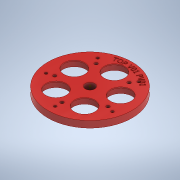
# Autodesk Inventor part: filterHolderBackPiece
Saved by Autodesk Inventor 2022.2 (Build 262287000, 287)
## iProperties
Created: 2020-04-12
Part Number: filterHolderBackPiece
Material: PBT Plastic
Document SubType Name: Modeling
Designer: robst
Density: 1.31 g/cm^3
Appearance: Orange-Red
wheelOuterDiameter: 4.501 in
wheelFilterDiameter: 2.611 in
filterThreadDiameter: 1.100 in
numberOfFilters: 5.000 ul
d5: 360.00 deg
distanceBetweenFilters: 0.500 in
distanceFromFilterToEdge: 0.375 in
wheelFilterCircumference: 8.200 in
filterDiameter: 1.140 in
Author: robst
Autodesk Inventor part; units mm, degrees
ref_plane "YZ Plane" through (0, 0, 0) normal (1, 0, 0) x (0, 1, 0)
ref_plane "XZ Plane" through (0, 0, 0) normal (0, 1, 0) x (-1, 0, 0)
ref_plane "XY Plane" through (0, 0, 0) normal (0, 0, 1) x (1, 0, 0)
sketch "Sketch1" plane through (0, 0, 0) normal (0, 1, 0) x (-1, 0, 0)
  circle A0 centre (0, 0) radius 57.1686
  circle A1 centre (0, 0) radius 33.1656 construction
  circle A2 centre (0, -33.1656) radius 13.97
  circle A3 centre (31.5424, -10.2487) radius 13.97
  circle A4 centre (19.4943, 26.8315) radius 13.97
  circle A5 centre (-19.4943, 26.8315) radius 13.97
  circle A6 centre (-31.5424, -10.2487) radius 13.97
  dimension "wheelFilterDiameter" = 66.3312
  dimension "wheelOuterDiameter" = 114.3372
  dimension "filterThreadDiameter" = 27.94
  dimension "d5" = 360
  constraints: 6 centre point, 2 coincident, 1 vertical alignment, 13 other
  measures "wheelOuterDiameter" diameter of A0
  measures "filterThreadDiameter" diameter of A2
extrude "Extrusion5" add sketch "Sketch1" against normal blind 8.89
sketch "Sketch5" plane through (0, 0, 0) normal (0, 1, 0) x (1, 0, 0)
  arc A0 (35.921, 35.921) -> (0, 50.8) centre (0, 0) ccw construction
  line L0 (0, 0) -> (0, 50.8) construction
  line L1 (0, 0) -> (35.921, 35.921) construction
  line L2 (0, 0) -> (50.8, 0) construction
  line L3 (-13.9692, 45.6649) -> (-15.4973, 50.8179)
  line L4 (-15.4973, 50.8179) -> (-17.4581, 50.2364)
  line L5 (-17.4581, 50.2364) -> (-17.6631, 50.9279)
  line L6 (-17.6631, 50.9279) -> (-12.9648, 52.3211)
  line L7 (-12.9648, 52.3211) -> (-12.7598, 51.6296)
  line L8 (-12.7598, 51.6296) -> (-14.7205, 51.0482)
  line L9 (-14.7205, 51.0482) -> (-13.1925, 45.8952)
  line L10 (-13.1925, 45.8952) -> (-13.9692, 45.6649)
  spline S0 degree 2 poles (-7.3189, 52.6818) (-6.9078, 52.3431) (-6.322, 51.2426) (-6.1896, 50.4935) knots 0 0 0 1 2 2 2
  spline S1 degree 2 poles (-6.1896, 50.4935) (-6.0606, 49.7638) (-6.2213, 48.5163) (-6.5011, 48.0555) knots 0 0 0 1 2 2 2
  spline S2 degree 2 poles (-6.5011, 48.0555) (-6.7968, 47.5718) (-7.7041, 47.0001) (-8.2927, 46.896) knots 0 0 0 1 2 2 2
  spline S3 degree 2 poles (-8.2927, 46.896) (-8.9008, 46.7885) (-9.9468, 47.03) (-10.3733, 47.371) knots 0 0 0 1 2 2 2
  spline S4 degree 2 poles (-10.3733, 47.371) (-10.7892, 47.7088) (-11.3662, 48.8158) (-11.4969, 49.5553) knots 0 0 0 1 2 2 2
  spline S5 degree 2 poles (-11.4969, 49.5553) (-11.6302, 50.3093) (-11.4585, 51.5235) (-11.1862, 51.9981) knots 0 0 0 1 2 2 2
  spline S6 degree 2 poles (-11.1862, 51.9981) (-10.9065, 52.4589) (-10.0018, 53.0452) (-9.3986, 53.1519) knots 0 0 0 1 2 2 2
  spline S7 degree 2 poles (-9.3986, 53.1519) (-8.7857, 53.2602) (-7.7273, 53.0059) (-7.3189, 52.6818) knots 0 0 0 1 2 2 2
  spline S8 degree 2 poles (-7.0214, 50.3464) (-7.1263, 50.9399) (-7.5467, 51.8137) (-7.8335, 52.0741) knots 0 0 0 1 2 2 2
  spline S9 degree 2 poles (-7.8335, 52.0741) (-8.1269, 52.3433) (-8.8533, 52.5359) (-9.2716, 52.462) knots 0 0 0 1 2 2 2
  spline S10 degree 2 poles (-9.2716, 52.462) (-9.7046, 52.3854) (-10.3031, 51.9686) (-10.4945, 51.6037) knots 0 0 0 1 2 2 2
  spline S11 degree 2 poles (-10.4945, 51.6037) (-10.6786, 51.2551) (-10.7682, 50.2861) (-10.665, 49.7023) knots 0 0 0 1 2 2 2
  spline S12 degree 2 poles (-10.665, 49.7023) (-10.4561, 48.5202) (-9.2418, 47.4406) (-8.41, 47.5876) knots 0 0 0 1 2 2 2
  spline S13 degree 2 poles (-8.41, 47.5876) (-7.5781, 47.7347) (-6.8125, 49.1643) (-7.0214, 50.3464) knots 0 0 0 1 2 2 2
  spline S14 degree 2 poles (-1.2006, 52.0412) (-1.1751, 51.6469) (-1.4102, 50.9188) (-1.6457, 50.6561) knots 0 0 0 1 2 2 2
  spline S15 degree 2 poles (-1.6457, 50.6561) (-1.9412, 50.3251) (-2.7733, 49.9495) (-3.424, 49.9075) knots 0 0 0 1 2 2 2
  line L11 (-3.424, 49.9075) -> (-4.1093, 49.8632)
  line L12 (-4.1093, 49.8632) -> (-3.9627, 47.5955)
  line L13 (-3.9627, 47.5955) -> (-4.7711, 47.5433)
  line L14 (-4.7711, 47.5433) -> (-5.1644, 53.6266)
  line L15 (-5.1644, 53.6266) -> (-3.6362, 53.7253)
  spline S16 degree 2 poles (-3.6362, 53.7253) (-3.0939, 53.7604) (-2.3232, 53.632) (-2.0193, 53.4487) knots 0 0 0 1 2 2 2
  spline S17 degree 2 poles (-2.0193, 53.4487) (-1.6642, 53.239) (-1.2335, 52.549) (-1.2006, 52.0412) knots 0 0 0 1 2 2 2
  spline S18 degree 2 poles (-2.042, 51.9621) (-2.0624, 52.2776) (-2.3093, 52.727) (-2.5407, 52.8605) knots 0 0 0 1 2 2 2
  spline S19 degree 2 poles (-2.5407, 52.8605) (-2.7412, 52.9763) (-3.2606, 53.0467) (-3.6402, 53.0221) knots 0 0 0 1 2 2 2
  line L16 (-3.6402, 53.0221) -> (-4.3106, 52.9788)
  line L17 (-4.3106, 52.9788) -> (-4.1539, 50.5534)
  line L18 (-4.1539, 50.5534) -> (-3.6017, 50.589)
  spline S20 degree 2 poles (-3.6017, 50.589) (-3.1088, 50.6209) (-2.5126, 50.8179) (-2.3288, 51.0377) knots 0 0 0 1 2 2 2
  spline S21 degree 2 poles (-2.3288, 51.0377) (-2.1582, 51.2318) (-2.0232, 51.6712) (-2.042, 51.9621) knots 0 0 0 1 2 2 2
  line L19 (7.4234, 53.3925) -> (4.7744, 47.5144)
  line L20 (4.7744, 47.5144) -> (3.9037, 47.5945)
  line L21 (3.9037, 47.5945) -> (2.3713, 53.8572)
  line L22 (2.3713, 53.8572) -> (3.2371, 53.7775)
  line L23 (3.2371, 53.7775) -> (4.4558, 48.5806)
  line L24 (4.4558, 48.5806) -> (6.6019, 53.4681)
  line L25 (6.6019, 53.4681) -> (7.4234, 53.3925)
  spline S22 degree 2 poles (11.6414, 49.4866) (11.3274, 47.8769) (10.0975, 46.5515) (9.1229, 46.7416) knots 0 0 0 1 2 2 2
  spline S23 degree 2 poles (9.1229, 46.7416) (8.1338, 46.9345) (7.5075, 48.6522) (7.8149, 50.228) knots 0 0 0 1 2 2 2
  spline S24 degree 2 poles (7.8149, 50.228) (8.1308, 51.8475) (9.3589, 53.1632) (10.3383, 52.9721) knots 0 0 0 1 2 2 2
  spline S25 degree 2 poles (10.3383, 52.9721) (11.3226, 52.7801) (11.946, 51.0479) (11.6414, 49.4866) knots 0 0 0 1 2 2 2
  spline S26 degree 2 poles (10.2579, 47.864) (10.432, 48.1371) (10.7067, 49.0297) (10.8269, 49.6455) knots 0 0 0 1 2 2 2
  spline S27 degree 2 poles (10.8269, 49.6455) (10.947, 50.2613) (11.0269, 51.1869) (10.9652, 51.516) knots 0 0 0 1 2 2 2
  spline S28 degree 2 poles (10.9652, 51.516) (10.9036, 51.8451) (10.5433, 52.2426) (10.2087, 52.3078) knots 0 0 0 1 2 2 2
  spline S29 degree 2 poles (10.2087, 52.3078) (9.8741, 52.3731) (9.3811, 52.1421) (9.1936, 51.8515) knots 0 0 0 1 2 2 2
  spline S30 degree 2 poles (9.1936, 51.8515) (9.0128, 51.5697) (8.7439, 50.6558) (8.6295, 50.0691) knots 0 0 0 1 2 2 2
  spline S31 degree 2 poles (8.6295, 50.0691) (8.5065, 49.4388) (8.4195, 48.58) (8.4813, 48.2257) knots 0 0 0 1 2 2 2
  spline S32 degree 2 poles (8.4813, 48.2257) (8.5371, 47.8927) (8.9034, 47.474) (9.2525, 47.4059) knots 0 0 0 1 2 2 2
  spline S33 degree 2 poles (9.2525, 47.4059) (9.5822, 47.3415) (10.0752, 47.5725) (10.2579, 47.864) knots 0 0 0 1 2 2 2
  line L26 (15.1243, 45.3222) -> (12.2732, 46.168)
  line L27 (12.2732, 46.168) -> (12.4502, 46.7647)
  line L28 (12.4502, 46.7647) -> (13.5111, 46.45)
  line L29 (13.5111, 46.45) -> (14.673, 50.3667)
  line L30 (14.673, 50.3667) -> (13.6121, 50.6814)
  line L31 (13.6121, 50.6814) -> (13.7708, 51.2166)
  spline S34 degree 2 poles (13.7708, 51.2166) (14.3723, 51.0382) (15.0418, 51.2106) (15.2202, 51.6729) knots 0 0 0 1 2 2 2
  line L32 (15.2202, 51.6729) -> (15.8264, 51.4931)
  line L33 (15.8264, 51.4931) -> (14.2641, 46.2266)
  line L34 (14.2641, 46.2266) -> (15.3013, 45.9189)
  line L35 (15.3013, 45.9189) -> (15.1243, 45.3222)
  spline S35 degree 2 poles (24.0801, 46.1507) (23.9119, 45.793) (23.3545, 45.269) (23.0214, 45.1527) knots 0 0 0 1 2 2 2
  spline S36 degree 2 poles (23.0214, 45.1527) (22.6029, 45.0055) (21.6928, 45.0785) (21.1027, 45.3559) knots 0 0 0 1 2 2 2
  line L36 (21.1027, 45.3559) -> (20.4813, 45.648)
  line L37 (20.4813, 45.648) -> (19.5145, 43.5915)
  line L38 (19.5145, 43.5915) -> (18.7813, 43.9362)
  line L39 (18.7813, 43.9362) -> (21.3747, 49.453)
  line L40 (21.3747, 49.453) -> (22.7606, 48.8015)
  spline S37 degree 2 poles (22.7606, 48.8015) (23.2524, 48.5703) (23.8652, 48.0857) (24.0428, 47.7785) knots 0 0 0 1 2 2 2
  spline S38 degree 2 poles (24.0428, 47.7785) (24.2525, 47.4233) (24.2965, 46.6111) (24.0801, 46.1507) knots 0 0 0 1 2 2 2
  spline S39 degree 2 poles (23.3051, 46.4877) (23.4396, 46.7738) (23.4404, 47.2865) (23.3023, 47.5152) knots 0 0 0 1 2 2 2
  spline S40 degree 2 poles (23.3023, 47.5152) (23.1825, 47.7134) (22.7617, 48.0259) (22.4175, 48.1877) knots 0 0 0 1 2 2 2
  line L41 (22.4175, 48.1877) -> (21.8095, 48.4735)
  line L42 (21.8095, 48.4735) -> (20.7755, 46.2739)
  line L43 (20.7755, 46.2739) -> (21.2762, 46.0385)
  spline S41 degree 2 poles (21.2762, 46.0385) (21.7233, 45.8284) (22.3404, 45.7129) (22.6075, 45.8167) knots 0 0 0 1 2 2 2
  spline S42 degree 2 poles (22.6075, 45.8167) (22.8507, 45.9043) (23.1811, 46.2239) (23.3051, 46.4877) knots 0 0 0 1 2 2 2
  line L44 (29.8707, 44.8732) -> (24.9322, 40.7284)
  line L45 (24.9322, 40.7284) -> (24.1826, 41.1786)
  line L46 (24.1826, 41.1786) -> (25.5215, 47.4855)
  line L47 (25.5215, 47.4855) -> (26.2669, 47.0378)
  line L48 (26.2669, 47.0378) -> (25.108, 41.8272)
  line L49 (25.108, 41.8272) -> (29.1635, 45.298)
  line L50 (29.1635, 45.298) -> (29.8707, 44.8732)
  spline S43 degree 2 poles (31.9744, 39.5232) (30.9925, 38.2095) (29.3091, 37.5496) (28.5137, 38.1441) knots 0 0 0 1 2 2 2
  spline S44 degree 2 poles (28.5137, 38.1441) (27.7065, 38.7474) (27.8882, 40.5666) (28.8493, 41.8526) knots 0 0 0 1 2 2 2
  spline S45 degree 2 poles (28.8493, 41.8526) (29.8371, 43.1743) (31.5146, 43.8262) (32.3139, 43.2288) knots 0 0 0 1 2 2 2
  spline S46 degree 2 poles (32.3139, 43.2288) (33.1172, 42.6285) (32.9267, 40.7974) (31.9744, 39.5232) knots 0 0 0 1 2 2 2
  spline S47 degree 2 poles (30.0235, 38.6624) (30.2989, 38.8328) (30.934, 39.5175) (31.3096, 40.0201) knots 0 0 0 1 2 2 2
  spline S48 degree 2 poles (31.3096, 40.0201) (31.6852, 40.5226) (32.1591, 41.3217) (32.2465, 41.6449) knots 0 0 0 1 2 2 2
  spline S49 degree 2 poles (32.2465, 41.6449) (32.3338, 41.9682) (32.1818, 42.4827) (31.9088, 42.6867) knots 0 0 0 1 2 2 2
  spline S50 degree 2 poles (31.9088, 42.6867) (31.6357, 42.8908) (31.0913, 42.8968) (30.7962, 42.7165) knots 0 0 0 1 2 2 2
  spline S51 degree 2 poles (30.7962, 42.7165) (30.511, 42.5411) (29.872, 41.8346) (29.5141, 41.3558) knots 0 0 0 1 2 2 2
  spline S52 degree 2 poles (29.5141, 41.3558) (29.1297, 40.8414) (28.6784, 40.1055) (28.5802, 39.7596) knots 0 0 0 1 2 2 2
  spline S53 degree 2 poles (28.5802, 39.7596) (28.4859, 39.4353) (28.634, 38.8991) (28.9189, 38.6862) knots 0 0 0 1 2 2 2
  spline S54 degree 2 poles (28.9189, 38.6862) (29.188, 38.4851) (29.7324, 38.4791) (30.0235, 38.6624) knots 0 0 0 1 2 2 2
  line L51 (33.3036, 34.2596) -> (31.1025, 36.2594)
  line L52 (31.1025, 36.2594) -> (31.5211, 36.7201)
  line L53 (31.5211, 36.7201) -> (32.3401, 35.976)
  line L54 (32.3401, 35.976) -> (35.0874, 38.9997)
  line L55 (35.0874, 38.9997) -> (34.2684, 39.7438)
  line L56 (34.2684, 39.7438) -> (34.6438, 40.157)
  spline S55 degree 2 poles (34.6438, 40.157) (35.1081, 39.7351) (35.786, 39.5997) (36.1475, 39.9388) knots 0 0 0 1 2 2 2
  line L57 (36.1475, 39.9388) -> (36.6155, 39.5136)
  line L58 (36.6155, 39.5136) -> (32.9214, 35.4478)
  line L59 (32.9214, 35.4478) -> (33.7221, 34.7203)
  line L60 (33.7221, 34.7203) -> (33.3036, 34.2596)
  dimension "d25" = 101.6
  dimension "d26" = 45
  constraints: 6 end point, 2 point on circle, 1 centre point, 1 coincident, 1 equal length, 1 horizontal, 1 vertical, 1 other
  measures "d25" diameter of A0
  measures "d26" angle of L2 L1
extrude "TextForTop" cut sketch "Sketch5" against normal blind 1.016
sketch "Sketch6" plane through (0, -8.89, 0) normal (0, -1, 0) x (1, 0, 0)
  circle A0 centre (19.4943, 26.8315) radius 13.97 projected
  circle A1 centre (19.4943, 26.8315) radius 15.621
  point P0 (0, 0)
  dimension "d29" = 31.242
  constraints: 1 centre point, 1 coincident
  measures "d29" diameter of A1
extrude "Extrusion7" cut sketch "Sketch6" against normal blind 7.62 contours A0 | A1
pattern_circular "Circular Pattern2" count 5 over 360 about axis through (0, -10, 0) along (0, 1, 0) of "Extrusion7"
sketch "Sketch7" plane through (0, 0, 0) normal (0, 1, 0) x (1, 0, 0)
  circle A0 centre (0, 0) radius 6.477
  dimension "d35" = 12.954
  constraints: 1 centre point, 1 coincident
  measures "d35" diameter of A0
extrude "Extrusion8" cut sketch "Sketch7" against normal through all
sketch "Sketch8" plane through (0, 0, 0) normal (0, 1, 0) x (1, 0, 0)
  circle A0 centre (0, 0) radius 47.1356 construction
  circle A1 centre (19.4943, -26.8315) radius 13.97 construction
  circle A2 centre (0, 0) radius 6.477 construction
  line L0 (0, 0) -> (27.7056, 38.1335) construction
  line L1 (0, 0) -> (0, 47.1356) construction
  circle A3 centre (0, 33.1656) radius 13.97 construction
  point P0 (-27.7056, 38.1335)
  point P1 (-44.8286, -14.5657)
  point P2 (0, -47.1356)
  point P3 (44.8286, -14.5657)
  dimension "d38" = 36
  dimension "d41" = 360
  constraints: 4 end point, 2 coincident, 2 point on circle, 1 centre point, 1 tangent, 1 vertical alignment, 7 other
  measures "d38" angle of L0 L1
sketch "Sketch10" plane through (0, -8.89, 0) normal (0, -1, 0) x (1, 0, 0)
  circle A0 centre (0, 0) radius 6.477 construction
  circle A1 centre (0, 0) radius 50.8 construction
  spline S0 degree 2 poles (-44.0461, 23.3584) (-43.705, 23.1938) (-43.3074, 22.6821) (-43.2405, 22.3847) knots 0 0 0 1 2 2 2
  spline S1 degree 2 poles (-43.2405, 22.3847) (-43.1655, 22.0286) (-43.2793, 21.3568) (-43.5047, 20.8896) knots 0 0 0 1 2 2 2
  line L0 (-43.5047, 20.8896) -> (-44.1379, 19.577)
  line L1 (-44.1379, 19.577) -> (-48.7134, 21.7841)
  line L2 (-48.7134, 21.7841) -> (-48.1285, 22.9966)
  spline S2 degree 2 poles (-48.1285, 22.9966) (-47.8924, 23.486) (-47.5933, 23.9451) (-47.3636, 24.1085) knots 0 0 0 1 2 2 2
  spline S3 degree 2 poles (-47.3636, 24.1085) (-47.114, 24.2943) (-46.5785, 24.3148) (-46.2893, 24.1753) knots 0 0 0 1 2 2 2
  spline S4 degree 2 poles (-46.2893, 24.1753) (-45.9667, 24.0197) (-45.6196, 23.4318) (-45.6198, 23.0617) knots 0 0 0 1 2 2 2
  line L3 (-45.6198, 23.0617) -> (-45.5976, 23.0509)
  spline S5 degree 2 poles (-45.5976, 23.0509) (-45.2896, 23.4052) (-44.4836, 23.5694) (-44.0461, 23.3584) knots 0 0 0 1 2 2 2
  spline S6 degree 2 poles (-44.326, 22.7118) (-44.5855, 22.837) (-44.9908, 22.8497) (-45.2168, 22.6844) knots 0 0 0 1 2 2 2
  spline S7 degree 2 poles (-45.2168, 22.6844) (-45.3607, 22.5756) (-45.5697, 22.2559) (-45.7217, 21.9408) knots 0 0 0 1 2 2 2
  line L4 (-45.7217, 21.9408) -> (-46.0544, 21.2511)
  line L5 (-46.0544, 21.2511) -> (-44.3636, 20.4355)
  line L6 (-44.3636, 20.4355) -> (-44.1258, 20.9287)
  spline S8 degree 2 poles (-44.1258, 20.9287) (-43.9326, 21.3291) (-43.785, 21.8246) (-43.8178, 22.0599) knots 0 0 0 1 2 2 2
  spline S9 degree 2 poles (-43.8178, 22.0599) (-43.8578, 22.2894) (-44.085, 22.5955) (-44.326, 22.7118) knots 0 0 0 1 2 2 2
  spline S10 degree 2 poles (-46.5098, 23.5001) (-46.673, 23.5788) (-46.9714, 23.5856) (-47.1008, 23.4973) knots 0 0 0 1 2 2 2
  spline S11 degree 2 poles (-47.1008, 23.4973) (-47.2539, 23.3883) (-47.4645, 23.0465) (-47.6201, 22.7239) knots 0 0 0 1 2 2 2
  line L7 (-47.6201, 22.7239) -> (-47.9009, 22.1418)
  line L8 (-47.9009, 22.1418) -> (-46.5624, 21.4961)
  line L9 (-46.5624, 21.4961) -> (-46.2297, 22.1858)
  spline S12 degree 2 poles (-46.2297, 22.1858) (-46.092, 22.4713) (-46.0208, 22.7706) (-46.0437, 22.9599) knots 0 0 0 1 2 2 2
  spline S13 degree 2 poles (-46.0437, 22.9599) (-46.0647, 23.1437) (-46.2948, 23.3964) (-46.5098, 23.5001) knots 0 0 0 1 2 2 2
  spline S14 degree 2 poles (-41.6038, 25.2552) (-41.5936, 25.1585) (-41.5492, 24.8272) (-41.5584, 24.6894) knots 0 0 0 1 2 2 2
  spline S15 degree 2 poles (-41.5584, 24.6894) (-41.5656, 24.498) (-41.6442, 24.1766) (-41.7899, 23.928) knots 0 0 0 1 2 2 2
  spline S16 degree 2 poles (-41.7899, 23.928) (-41.9085, 23.7255) (-42.2756, 23.4492) (-42.4953, 23.3919) knots 0 0 0 1 2 2 2
  spline S17 degree 2 poles (-42.4953, 23.3919) (-42.7073, 23.3395) (-43.1987, 23.4128) (-43.4189, 23.5419) knots 0 0 0 1 2 2 2
  spline S18 degree 2 poles (-43.4189, 23.5419) (-43.7599, 23.7417) (-44.0744, 24.3124) (-44.0297, 24.7061) knots 0 0 0 1 2 2 2
  spline S19 degree 2 poles (-44.0297, 24.7061) (-43.9953, 25.0581) (-43.6499, 25.8673) (-43.4188, 26.3187) knots 0 0 0 1 2 2 2
  line L10 (-43.4188, 26.3187) -> (-43.5253, 26.3812)
  spline S20 degree 2 poles (-43.5253, 26.3812) (-43.7171, 26.4936) (-44.0238, 26.5158) (-44.1537, 26.4488) knots 0 0 0 1 2 2 2
  spline S21 degree 2 poles (-44.1537, 26.4488) (-44.2836, 26.3818) (-44.5052, 26.1013) (-44.601, 25.9379) knots 0 0 0 1 2 2 2
  spline S22 degree 2 poles (-44.601, 25.9379) (-44.7134, 25.7461) (-44.9036, 25.161) (-44.9454, 24.8372) knots 0 0 0 1 2 2 2
  line L11 (-44.9454, 24.8372) -> (-44.9642, 24.8052)
  line L12 (-44.9642, 24.8052) -> (-45.5289, 25.1361)
  spline S23 degree 2 poles (-45.5289, 25.1361) (-45.482, 25.3138) (-45.2535, 25.9481) (-45.0891, 26.2287) knots 0 0 0 1 2 2 2
  spline S24 degree 2 poles (-45.0891, 26.2287) (-44.8892, 26.5697) (-44.51, 26.9725) (-44.2633, 27.076) knots 0 0 0 1 2 2 2
  spline S25 degree 2 poles (-44.2633, 27.076) (-44.0222, 27.1781) (-43.4883, 27.1038) (-43.1793, 26.9228) knots 0 0 0 1 2 2 2
  line L13 (-43.1793, 26.9228) -> (-40.931, 25.6053)
  line L14 (-40.931, 25.6053) -> (-41.2557, 25.0512)
  line L15 (-41.2557, 25.0512) -> (-41.6038, 25.2552)
  line L16 (-42.0655, 25.5257) -> (-42.9784, 26.0606)
  spline S26 degree 2 poles (-42.9784, 26.0606) (-43.0771, 25.8513) (-43.3685, 25.2157) (-43.422, 24.9942) knots 0 0 0 1 2 2 2
  spline S27 degree 2 poles (-43.422, 24.9942) (-43.4836, 24.7344) (-43.3716, 24.2823) (-43.1229, 24.1366) knots 0 0 0 1 2 2 2
  spline S28 degree 2 poles (-43.1229, 24.1366) (-42.8388, 23.9701) (-42.3638, 24.1212) (-42.1848, 24.4266) knots 0 0 0 1 2 2 2
  spline S29 degree 2 poles (-42.1848, 24.4266) (-42.0328, 24.6859) (-42.0068, 25.2432) (-42.0655, 25.5257) knots 0 0 0 1 2 2 2
  spline S30 degree 2 poles (-39.5121, 27.5613) (-39.7357, 27.2354) (-40.3063, 26.8331) (-40.6427, 26.7794) knots 0 0 0 1 2 2 2
  spline S31 degree 2 poles (-40.6427, 26.7794) (-40.9758, 26.7234) (-41.7403, 26.9335) (-42.1544, 27.2176) knots 0 0 0 1 2 2 2
  spline S32 degree 2 poles (-42.1544, 27.2176) (-42.5685, 27.5018) (-43.0213, 28.1371) (-43.0968, 28.4635) knots 0 0 0 1 2 2 2
  spline S33 degree 2 poles (-43.0968, 28.4635) (-43.1758, 28.7923) (-43.0167, 29.497) (-42.7978, 29.816) knots 0 0 0 1 2 2 2
  spline S34 degree 2 poles (-42.7978, 29.816) (-42.6208, 30.074) (-42.144, 30.4558) (-41.9209, 30.5773) knots 0 0 0 1 2 2 2
  line L17 (-41.9209, 30.5773) -> (-41.3269, 30.1697)
  line L18 (-41.3269, 30.1697) -> (-41.3478, 30.1391)
  spline S35 degree 2 poles (-41.3478, 30.1391) (-41.435, 30.114) (-41.6783, 30.0214) (-41.829, 29.94) knots 0 0 0 1 2 2 2
  spline S36 degree 2 poles (-41.829, 29.94) (-41.9601, 29.8653) (-42.25, 29.6248) (-42.3431, 29.4891) knots 0 0 0 1 2 2 2
  spline S37 degree 2 poles (-42.3431, 29.4891) (-42.625, 29.0783) (-42.3462, 28.1531) (-41.7794, 27.7641) knots 0 0 0 1 2 2 2
  spline S38 degree 2 poles (-41.7794, 27.7641) (-41.2261, 27.3844) (-40.2742, 27.4402) (-39.9807, 27.8679) knots 0 0 0 1 2 2 2
  spline S39 degree 2 poles (-39.9807, 27.8679) (-39.8037, 28.1258) (-39.6961, 28.741) (-39.7389, 29.035) knots 0 0 0 1 2 2 2
  line L19 (-39.7389, 29.035) -> (-39.718, 29.0656)
  line L20 (-39.718, 29.0656) -> (-39.124, 28.658)
  spline S40 degree 2 poles (-39.124, 28.658) (-39.1402, 28.5543) (-39.198, 28.2445) (-39.2395, 28.1331) knots 0 0 0 1 2 2 2
  spline S41 degree 2 poles (-39.2395, 28.1331) (-39.2919, 27.9694) (-39.3979, 27.7276) (-39.5121, 27.5613) knots 0 0 0 1 2 2 2
  line L21 (-36.6315, 31.4756) -> (-37.1561, 30.8145)
  line L22 (-37.1561, 30.8145) -> (-39.4778, 30.8492)
  line L23 (-39.4778, 30.8492) -> (-39.443, 30.4957)
  line L24 (-39.443, 30.4957) -> (-38.1951, 29.5053)
  line L25 (-38.1951, 29.5053) -> (-38.5943, 29.0023)
  line L26 (-38.5943, 29.0023) -> (-42.7508, 32.301)
  line L27 (-42.7508, 32.301) -> (-42.3516, 32.804)
  line L28 (-42.3516, 32.804) -> (-39.9202, 30.8744)
  line L29 (-39.9202, 30.8744) -> (-40.2444, 33.0553)
  line L30 (-40.2444, 33.0553) -> (-39.748, 33.6808)
  line L31 (-39.748, 33.6808) -> (-39.4725, 31.4651)
  line L32 (-39.4725, 31.4651) -> (-36.6315, 31.4756)
  line L33 (-35.8317, 39.5676) -> (-33.5272, 34.714)
  line L34 (-33.5272, 34.714) -> (-34.0478, 34.2042)
  line L35 (-34.0478, 34.2042) -> (-38.8522, 36.6094)
  line L36 (-38.8522, 36.6094) -> (-38.3346, 37.1164)
  line L37 (-38.3346, 37.1164) -> (-34.3763, 35.0868)
  line L38 (-34.3763, 35.0868) -> (-36.3228, 39.0866)
  line L39 (-36.3228, 39.0866) -> (-35.8317, 39.5676)
  spline S42 degree 2 poles (-31.1508, 40.1611) (-30.279, 39.1085) (-30.0742, 37.6157) (-30.7115, 37.0879) knots 0 0 0 1 2 2 2
  spline S43 degree 2 poles (-30.7115, 37.0879) (-31.3583, 36.5522) (-32.7962, 37.0557) (-33.6496, 38.0861) knots 0 0 0 1 2 2 2
  spline S44 degree 2 poles (-33.6496, 38.0861) (-34.5267, 39.1451) (-34.7262, 40.6316) (-34.0857, 41.162) knots 0 0 0 1 2 2 2
  spline S45 degree 2 poles (-34.0857, 41.162) (-33.4421, 41.695) (-31.9963, 41.182) (-31.1508, 40.1611) knots 0 0 0 1 2 2 2
  spline S46 degree 2 poles (-30.8356, 38.4123) (-30.9197, 38.6687) (-31.3499, 39.3173) (-31.6834, 39.72) knots 0 0 0 1 2 2 2
  spline S47 degree 2 poles (-31.6834, 39.72) (-32.0169, 40.1226) (-32.5713, 40.663) (-32.816, 40.7971) knots 0 0 0 1 2 2 2
  spline S48 degree 2 poles (-32.816, 40.7971) (-33.0607, 40.9312) (-33.5072, 40.9088) (-33.726, 40.7276) knots 0 0 0 1 2 2 2
  spline S49 degree 2 poles (-33.726, 40.7276) (-33.9448, 40.5464) (-34.0562, 40.1067) (-33.968, 39.8323) knots 0 0 0 1 2 2 2
  spline S50 degree 2 poles (-33.968, 39.8323) (-33.8818, 39.5669) (-33.4347, 38.9109) (-33.117, 38.5273) knots 0 0 0 1 2 2 2
  spline S51 degree 2 poles (-33.117, 38.5273) (-32.7756, 38.1151) (-32.268, 37.6055) (-32.007, 37.4581) knots 0 0 0 1 2 2 2
  spline S52 degree 2 poles (-32.007, 37.4581) (-31.7629, 37.3183) (-31.2995, 37.3332) (-31.0712, 37.5223) knots 0 0 0 1 2 2 2
  spline S53 degree 2 poles (-31.0712, 37.5223) (-30.8557, 37.7008) (-30.7442, 38.1406) (-30.8356, 38.4123) knots 0 0 0 1 2 2 2
  line L40 (-26.6579, 40.2515) -> (-28.6852, 38.8262)
  line L41 (-28.6852, 38.8262) -> (-28.9836, 39.2506)
  line L42 (-28.9836, 39.2506) -> (-28.2292, 39.7809)
  line L43 (-28.2292, 39.7809) -> (-30.1872, 42.566)
  line L44 (-30.1872, 42.566) -> (-30.9416, 42.0356)
  line L45 (-30.9416, 42.0356) -> (-31.2091, 42.4162)
  spline S54 degree 2 poles (-31.2091, 42.4162) (-30.7814, 42.7169) (-30.5478, 43.2435) (-30.7576, 43.5992) knots 0 0 0 1 2 2 2
  line L46 (-30.7576, 43.5992) -> (-30.3265, 43.9023)
  line L47 (-30.3265, 43.9023) -> (-27.6937, 40.1574)
  line L48 (-27.6937, 40.1574) -> (-26.9562, 40.6759)
  line L49 (-26.9562, 40.6759) -> (-26.6579, 40.2515)
  spline S55 degree 2 poles (-22.7106, 46.6004) (-22.5562, 46.3095) (-22.4854, 45.6759) (-22.5742, 45.3956) knots 0 0 0 1 2 2 2
  spline S56 degree 2 poles (-22.5742, 45.3956) (-22.6853, 45.043) (-23.1888, 44.4726) (-23.6687, 44.2178) knots 0 0 0 1 2 2 2
  line L50 (-23.6687, 44.2178) -> (-24.1741, 43.9494)
  line L51 (-24.1741, 43.9494) -> (-23.2859, 42.2769)
  line L52 (-23.2859, 42.2769) -> (-23.8822, 41.9603)
  line L53 (-23.8822, 41.9603) -> (-26.2648, 46.4468)
  line L54 (-26.2648, 46.4468) -> (-25.1377, 47.0454)
  spline S57 degree 2 poles (-25.1377, 47.0454) (-24.7378, 47.2578) (-24.1084, 47.4242) (-23.8147, 47.3891) knots 0 0 0 1 2 2 2
  spline S58 degree 2 poles (-23.8147, 47.3891) (-23.4731, 47.3514) (-22.9095, 46.9749) (-22.7106, 46.6004) knots 0 0 0 1 2 2 2
  spline S59 degree 2 poles (-23.3227, 46.252) (-23.4463, 46.4847) (-23.7877, 46.7415) (-24.0093, 46.7637) knots 0 0 0 1 2 2 2
  spline S60 degree 2 poles (-24.0093, 46.7637) (-24.2013, 46.7829) (-24.6199, 46.6585) (-24.8999, 46.5098) knots 0 0 0 1 2 2 2
  line L55 (-24.8999, 46.5098) -> (-25.3944, 46.2472)
  line L56 (-25.3944, 46.2472) -> (-24.4444, 44.4584)
  line L57 (-24.4444, 44.4584) -> (-24.0372, 44.6746)
  spline S61 degree 2 poles (-24.0372, 44.6746) (-23.6736, 44.8677) (-23.2882, 45.2216) (-23.2239, 45.4515) knots 0 0 0 1 2 2 2
  spline S62 degree 2 poles (-23.2239, 45.4515) (-23.1608, 45.6575) (-23.2088, 46.0375) (-23.3227, 46.252) knots 0 0 0 1 2 2 2
  line L58 (-19.0761, 49.8558) -> (-18.6852, 44.4972)
  line L59 (-18.6852, 44.4972) -> (-19.355, 44.2105)
  line L60 (-19.355, 44.2105) -> (-22.9627, 48.1919)
  line L61 (-22.9627, 48.1919) -> (-22.2967, 48.4771)
  line L62 (-22.2967, 48.4771) -> (-19.3417, 45.1521)
  line L63 (-19.3417, 45.1521) -> (-19.7081, 49.5853)
  line L64 (-19.7081, 49.5853) -> (-19.0761, 49.8558)
  spline S63 degree 2 poles (-14.4979, 48.7144) (-14.0663, 47.4176) (-14.4159, 45.9519) (-15.201, 45.6907) knots 0 0 0 1 2 2 2
  spline S64 degree 2 poles (-15.201, 45.6907) (-15.9979, 45.4255) (-17.156, 46.4154) (-17.5785, 47.6849) knots 0 0 0 1 2 2 2
  spline S65 degree 2 poles (-17.5785, 47.6849) (-18.0126, 48.9895) (-17.6604, 50.4474) (-16.8714, 50.71) knots 0 0 0 1 2 2 2
  spline S66 degree 2 poles (-16.8714, 50.71) (-16.0785, 50.9739) (-14.9164, 49.9722) (-14.4979, 48.7144) knots 0 0 0 1 2 2 2
  spline S67 degree 2 poles (-14.8372, 46.9702) (-14.8227, 47.2396) (-14.989, 48) (-15.1541, 48.4961) knots 0 0 0 1 2 2 2
  spline S68 degree 2 poles (-15.1541, 48.4961) (-15.3192, 48.9921) (-15.6404, 49.6966) (-15.8199, 49.9101) knots 0 0 0 1 2 2 2
  spline S69 degree 2 poles (-15.8199, 49.9101) (-15.9995, 50.1237) (-16.4238, 50.2645) (-16.6933, 50.1748) knots 0 0 0 1 2 2 2
  spline S70 degree 2 poles (-16.6933, 50.1748) (-16.9628, 50.0851) (-17.226, 49.7156) (-17.243, 49.4279) knots 0 0 0 1 2 2 2
  spline S71 degree 2 poles (-17.243, 49.4279) (-17.2588, 49.1493) (-17.0795, 48.3759) (-16.9222, 47.9033) knots 0 0 0 1 2 2 2
  spline S72 degree 2 poles (-16.9222, 47.9033) (-16.7533, 47.3955) (-16.4646, 46.7366) (-16.2746, 46.5048) knots 0 0 0 1 2 2 2
  spline S73 degree 2 poles (-16.2746, 46.5048) (-16.0977, 46.286) (-15.6603, 46.1322) (-15.3791, 46.2258) knots 0 0 0 1 2 2 2
  spline S74 degree 2 poles (-15.3791, 46.2258) (-15.1135, 46.3142) (-14.8503, 46.6838) (-14.8372, 46.9702) knots 0 0 0 1 2 2 2
  line L65 (-10.0293, 47.2334) -> (-13.0705, 46.4817)
  line L66 (-13.0705, 46.4817) -> (-13.2434, 47.1811)
  spline S75 degree 2 poles (-13.2434, 47.1811) (-12.9918, 47.5698) (-12.5495, 48.2855) (-12.3458, 48.6624) knots 0 0 0 1 2 2 2
  spline S76 degree 2 poles (-12.3458, 48.6624) (-11.9354, 49.4211) (-11.7075, 50.2662) (-11.8053, 50.6618) knots 0 0 0 1 2 2 2
  spline S77 degree 2 poles (-11.8053, 50.6618) (-11.8567, 50.8696) (-12.0616, 51.1497) (-12.2022, 51.221) knots 0 0 0 1 2 2 2
  spline S78 degree 2 poles (-12.2022, 51.221) (-12.3428, 51.2923) (-12.6712, 51.3171) (-12.8551, 51.2717) knots 0 0 0 1 2 2 2
  spline S79 degree 2 poles (-12.8551, 51.2717) (-13.0309, 51.2282) (-13.3689, 51.0514) (-13.5159, 50.9429) knots 0 0 0 1 2 2 2
  spline S80 degree 2 poles (-13.5159, 50.9429) (-13.642, 50.8524) (-13.8622, 50.6284) (-13.9283, 50.5526) knots 0 0 0 1 2 2 2
  line L67 (-13.9283, 50.5526) -> (-13.9643, 50.5438)
  line L68 (-13.9643, 50.5438) -> (-14.1381, 51.2471)
  spline S81 degree 2 poles (-14.1381, 51.2471) (-13.959, 51.3974) (-13.2761, 51.774) (-12.9484, 51.855) knots 0 0 0 1 2 2 2
  spline S82 degree 2 poles (-12.9484, 51.855) (-12.257, 52.0259) (-11.2969, 51.4872) (-11.1428, 50.8637) knots 0 0 0 1 2 2 2
  spline S83 degree 2 poles (-11.1428, 50.8637) (-11.0707, 50.572) (-11.0861, 50.0508) (-11.1546, 49.8134) knots 0 0 0 1 2 2 2
  spline S84 degree 2 poles (-11.1546, 49.8134) (-11.2212, 49.5679) (-11.4641, 49.0584) (-11.6056, 48.8072) knots 0 0 0 1 2 2 2
  spline S85 degree 2 poles (-11.6056, 48.8072) (-11.8334, 48.3904) (-12.4169, 47.4744) (-12.5923, 47.2063) knots 0 0 0 1 2 2 2
  line L69 (-12.5923, 47.2063) -> (-10.1705, 47.8049)
  line L70 (-10.1705, 47.8049) -> (-10.0293, 47.2334)
  dimension "d50" = 101.6
  constraints: 1 centre point, 1 coincident, 1 other
  measures "d50" diameter of A1
extrude "TextForBack" cut sketch "Sketch10" against normal blind 1.27
sketch "Sketch12" plane through (0, -8.89, 0) normal (0, -1, 0) x (1, 0, 0)
  circle A0 centre (0, 0) radius 38.1 construction
  line L0 (0, 0) -> (-36.2353, 11.7735) construction
  circle A1 centre (-31.5424, -10.2487) radius 15.621 construction
  circle A2 centre (-19.4943, 26.8315) radius 15.621 construction
  line L1 (-36.2353, 11.7735) -> (-37.8867, 4.0259) construction
  line L2 (-36.2353, 11.7735) -> (-33.0173, 19.0122) construction
  circle A3 centre (-19.4943, 26.8315) radius 15.621 construction
  point P0 (-22.3946, -30.8235)
  point P1 (22.3946, -30.8235)
  point P2 (36.2353, 11.7735)
  point P3 (0, 38.1)
  dimension "d54" = 76.2
  dimension "d57" = 360
  constraints: 6 end point, 3 point on circle, 2 coincident, 1 centre point, 1 equal length, 10 other
  measures "d54" diameter of A0
hole "Hole2" at (-36.2353, -8.89, 11.7735) at (-22.3946, -8.89, -30.8235) at (22.3946, -8.89, -30.8235) at (36.2353, -8.89, 11.7735) at (0, -8.89, 38.1) direction (0, 1, 0) diameter 4.4958 end through all clearance for "Flat Head Machine Screw (82)" size "#8" standard "Ansi Unified Screw Threads"
sketch "Sketch13" plane through (0, -8.89, 0) normal (0, -1, 0) x (1, 0, 0)
  circle A0 centre (0, 0) radius 57.1686 projected
  circle A1 centre (0, 0) radius 47.4531 construction
  point P0 (0, 47.4531)
  point P1 (-45.1306, 14.6638)
  point P2 (-27.8922, -38.3904)
  point P3 (27.8922, -38.3904)
  point P4 (45.1306, 14.6638)
  dimension "d67" = 9.7155
  dimension "d70" = 360
  constraints: 1 coincident, 1 vertical alignment, 8 other
hole "Hole3" at (0, -8.89, 47.4531) at (-45.1306, -8.89, 14.6638) at (-27.8922, -8.89, -38.3904) at (27.8922, -8.89, -38.3904) at (45.1306, -8.89, 14.6638) direction (0, 1, 0) diameter 3.81 end through all clearance for "Hex Machine Screw" size "#6" standard "Ansi Unified Screw Threads"
hole "Hole4" at (0, -8.89, 47.4531) at (45.1306, -8.89, 14.6638) at (27.8922, -8.89, -38.3904) at (-27.8922, -8.89, -38.3904) at (-45.1306, -8.89, 14.6638) direction (0, 1, 0) diameter 4.699 depth 7.0739 counterbore diameter 5.5372 counterbore depth 5.5524
equation "\"wheelFilterDiameter\" = 0.318471 * wheelFilterCircumference"
equation "\"wheelOuterDiameter\" = filterDiameter + wheelFilterDiameter + 2 * distanceFromFilterToEdge"
equation "\"d23\" = filterWheelThickness"
equation "\"d27\" = textDepth"
equation "\"d29\" = filterMaxDiameter"
equation "\"d30\" = filterDepth"
equation "\"d35\" = centerHoleDiameter"
equation "\"distanceBetweenFilters\" = 12.7"
equation "\"distanceFromFilterToEdge\" = 9.525"
equation "\"filterDiameter\" = 28.956"
equation "\"filterWheelThickness\" = 8.89"
equation "\"textDepth\" = 1.016"
equation "\"filterMaxDiameter\" = 31.242"
equation "\"filterDepth\" = 7.62"
equation "\"centerHoleDiameter\" = 12.954"
equation "\"eyepieceDiameter\" = 31.75"
equation "\"wheelFilterCircumference\" = 208.28"
body "Solid3"
